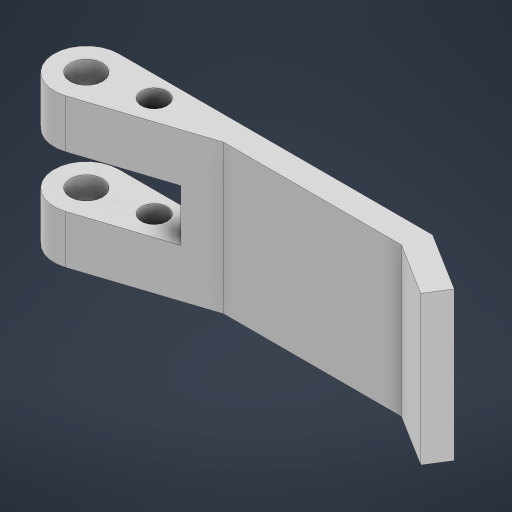
# Autodesk Inventor part: Lever
Saved by Autodesk Inventor 2024.2 (Build 282272000, 272)
## iProperties
Created: 2024-06-05
Part Number: Lever
Material: Generic
Document SubType Name: Modeling
Designer: simon
Density: 1 g/cm^3
Appearance: Default
Author: simon
Autodesk Inventor part; units mm, degrees
ref_plane "YZ Plane" through (0, 0, 0) normal (1, 0, 0) x (0, 1, 0)
ref_plane "XZ Plane" through (0, 0, 0) normal (0, 1, 0) x (-1, 0, 0)
ref_plane "XY Plane" through (0, 0, 0) normal (0, 0, 1) x (1, 0, 0)
sketch "Sketch1" plane through (0, 0, 0) normal (0, 0, 1) x (1, 0, 0)
  line L0 (0, 0) -> (50, 0)
  line L1 (50, 0) -> (50, 18.4)
  line L2 (50, 18.4) -> (0, 18.4)
  line L3 (0, 18.4) -> (0, 0)
  line L4 (0, 12.4) -> (16, 12.4)
  line L5 (16, 12.4) -> (16, 6)
  line L6 (16, 6) -> (0, 6)
  line L7 (0, 6) -> (0, 12.4)
  line L8 (58.8783, 9.2) -> (-7.6234, 9.2)
  point P0 (0, 6)
  dimension "d0" = 50
  dimension "d1" = 18.4
  dimension "d11" = 16
  dimension "d13" = 18.4
  dimension "d14" = 6.4
  dimension "d15" = 6.4
  constraints: 18 end point, 4 parallel, 3 horizontal, 2 perpendicular, 1 point on line
  measures "d0" distance of L2.end L1.end
  measures "d1" distance of L1.end L0.end
  measures "d11" distance of L5.end L6.end
  measures "d13" diameter of L2 L8
  measures "d14" diameter of L4 L8
  measures "d15" distance of L4.end L5.end
extrude "Extrusion1" add sketch "Sketch1" along normal blind 8 contours L3 L6 L5 L8 L1 L0 | L8 L5 L4 L3 L2 L1
fillet "Fillet1" radius 4 4 edges at (0, 3, 8) (0, 3, 0) (0, 15.4, 8) (0, 15.4, 0)
sketch "Sketch3" plane through (50, 0, 0) normal (0, -1, 0) x (1, 0, 0)
  circle A0 centre (-46, 4) radius 2
  line L0 (-46, 8) -> (0, 8) projected
  arc A1 (-46, 8) -> (-46, 0) centre (-46, 4) ccw projected
  circle A2 centre (-39, 2.6) radius 1.6
  line L1 (-46, 0) -> (0, 0) projected
  circle A3 centre (-46, 4) radius 4
  line L2 (-44.7623, 7.8037) -> (-30, 3)
  line L3 (-30, 3) -> (-8, 3)
  line L4 (-8, 3) -> (0, 8)
  line L5 (0, 0) -> (0, 8) projected
  line L6 (-7.1396, 0) -> (0, 4.4623)
  line L7 (0, 4.4623) -> (-1.59, 7.0063)
  point P0 (-50, 0)
  point P1 (-50, 4)
  point P2 (-50, 4)
  point P3 (-50, 4)
  point P4 (-4, 5.5)
  dimension "d23" = 8
  dimension "d17" = 4
  dimension "d18" = 4
  dimension "d19" = 4
  dimension "d20" = 3.2
  dimension "d21" = 2.6
  dimension "d22" = 11
  dimension "d24" = 20
  dimension "d25" = 8
  dimension "d26" = 5
  dimension "d27" = 3
  constraints: 10 end point, 3 point on circle, 3 point on line, 2 centre point, 1 coincident, 1 horizontal, 1 midpoint, 1 parallel, 1 perpendicular, 4 other
  measures "d17" diameter of A0
  measures "d18" distance from line of L0 A0.centre
  measures "d19" distance of point (-50, 4) A0.centre
  measures "d20" diameter of A2
  measures "d21" distance from line of A2.centre L1
  measures "d22" horizontal distance of point (-50, 4) A2.centre
  measures "d24" horizontal distance of point (-50, 4) L2.end
  measures "d25" distance from line of L3.end L5
  measures "d26" distance between parallel lines of L0 L3
  measures "d27" distance from line of point (-4, 5.5) L6
extrude "Extrusion3" cut sketch "Sketch3" against normal blind 20 contours A0 | L0 L4 L3 L2 A3 | L5 L7 L4 | L5 L1 L6 | A2
body "Solid1"
